# Autodesk Inventor part: BS 3692 - M30
Saved by Autodesk Inventor 2020.1 (Build 241239000, 239)
## iProperties
Comments: To add or edit properties for Autodesk Inventor files, use iProperties.
Shininess: 64.0
Length Units: 11269
Angle Units: 11279
Time Units: 11290
Mass Units: 11283
Length Display Precision: 3
Angle Display Precision: 2
Compacted: True
Alert: To add or edit properties for Autodesk Inventor files, use iProperties.
Created: 2003-05-03
Part Number: BS 3692 - M30
Vendor: Autodesk Inc.
Document SubType Name: Modeling
Designer: Stephen Hooper
Material: Generic
Description: Hex Nut
Standard: BS 3692
Manufacturer: Standard
Standards Organization: Custom
Density: 1 g/cm^3
Appearance: Default
Density: 0.0
Volumn: 0.0
Area: 0.0
PropertySet Name: Model Information
Control State: 0
Master: False
Checked Out: False
EGR: 1
Author: Stephen Hooper
Revision Number: 5
Autodesk Inventor part; units mm, degrees
ref_plane "YZ Plane" through (0, 0, 0) normal (1, 0, 0) x (0, 1, 0)
ref_plane "XZ Plane" through (0, 0, 0) normal (0, 1, 0) x (-1, 0, 0)
ref_plane "XY Plane" through (0, 0, 0) normal (0, 0, 1) x (1, 0, 0)
sketch "Sketch1" plane through (0, 0, 0) normal (1, 0, 0) x (0, 1, 0)
  line L0 (-26.5581, 0) -> (-13.2791, 23)
  line L1 (-13.2791, 23) -> (13.2791, 23)
  line L2 (13.2791, 23) -> (26.5581, 0)
  line L3 (26.5581, 0) -> (13.2791, -23)
  line L4 (13.2791, -23) -> (-13.2791, -23)
  line L5 (-13.2791, -23) -> (-26.5581, 0)
  point P0 (0, 0)
  point P1 (0, 0)
  dimension "d0" = 53.1162
  constraints: 12 end point, 1 coincident, 1 horizontal, 11 other
  measures "d0" distance of L2.end L0.start
extrude "Body" add sketch "Sketch1" along normal blind 24
sketch "Sketch2" plane through (0, 0, 0) normal (0, 0, 1) x (1, 0, 0)
  line L0 (0, 13.2791) -> (0, 26.5581) projected
  line L1 (0, 26.5581) -> (24, 26.5581) projected
  line L2 (24, 13.2791) -> (24, 26.5581) projected
  line L3 (-2.4, 0) -> (31.2, 0) projected
  line L4 (2.0543, 26.5581) -> (0, 23)
  line L5 (21.9457, 26.5581) -> (24, 23)
  dimension "d3" = 30
  dimension "d4" = 30
  dimension "d5" = 46
  dimension "d6" = 46
  constraints: 4 end point, 4 point on line
  measures "d3" angle of L0 L4
  measures "d4" angle of L2 L5
  measures "d5" diameter of L4.end L3
  measures "d6" diameter of L5.end L3
revolve "Chamfer1" cut sketch "Sketch2" angle 360 about axis through (-10, 0, 0) along (1, 0, 0)
sketch "Sketch3" plane through (24, 0, 0) normal (1, 0, 0) x (0, 0, -1)
  arc A0 (-11.5, -19.9186) -> (11.5, -19.9186) centre (0, 0) ccw projected
  constraints: 1 coincident
hole "Thread" at (24, 0, 0) direction (-1, 0, 0) diameter 26.211 end through all thread size "M30x3.5" class "6H" standard "ISO Metric profile"
chamfer "Chamfer2" distance 1.8944 angle 30 1 edges at (24, 0, 13.1055) measured on face at (24, 19.586, -0.5266)
chamfer "Chamfer3" distance 1.8944 angle 30 1 edges at (0, 0, 13.1055) measured on face at (0, 19.586, -0.5266)
equation "\"d0\" = 1.1547 * SW"
equation "\"d1\" = KOH"
equation "\"d3\" = ANG1"
equation "\"d4\" = ANG2"
equation "\"d5\" = SW0"
equation "\"d6\" = SW01"
equation "\"d8\" = -0.5 * GD1 + 0.5 * NND"
equation "\"d40\" = -0.5 * GD1 + 0.5 * NND"
equation "\"d10\" = -0.5 * GD1 + 0.5 * NND"
equation "\"d41\" = -0.5 * GD1 + 0.5 * NND"
equation "\"ANG1\" = 30deg"
equation "\"ANG2\" = ANG1"
equation "\"KOH\" = 24"
equation "\"SW\" = 46"
equation "\"SW0\" = SW"
equation "\"SW01\" = SW"
equation "\"TOA\" = 30deg"
equation "\"PTC\" = TPU"
equation "\"GAL\" = 0.541266 * TPU"
equation "\"GUL\" = 0.541266 * TPU"
equation "\"TPU\" = 3.5"
equation "\"E0\" = 1.155 * SW"
equation "\"GD1\" = 26.211139"
equation "\"NND\" = 30"
body "Solid1"
